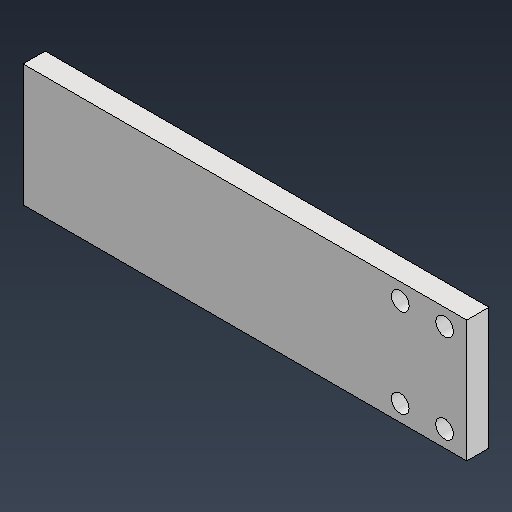
# Autodesk Inventor part: PLATE,HINGE,FRONT,INTAKE
Saved by Autodesk Inventor 2026 (Build 300175050, 175E)
## iProperties
Created: 2026-02-16
Part Number: PLATE,HINGE,FRONT,INTAKE
Material: Generic
Document SubType Name: Modeling
Designer: Jthib
Mass: 27.6453 g
Surface Area: 111.71 cm^2
Volume: 27.6453 cm^3
Density: 1 g/cm^3
Appearance: Default
Author: Jthib
Autodesk Inventor part; units mm, degrees
ref_plane "YZ Plane" through (0, 0, 0) normal (1, 0, 0) x (0, 1, 0)
ref_plane "XZ Plane" through (0, 0, 0) normal (0, 1, 0) x (-1, 0, 0)
ref_plane "XY Plane" through (0, 0, 0) normal (0, 0, 1) x (1, 0, 0)
sketch "Sketch1" plane through (0, 0, 0) normal (0, 0, 1) x (1, 0, 0)
  line L0 (63.5, -17.4625) -> (-63.5, -17.4625)
  line L1 (-63.5, -17.4625) -> (-63.5, 17.4625)
  line L2 (-63.5, 17.4625) -> (63.5, 17.4625)
  line L3 (63.5, 17.4625) -> (63.5, -17.4625)
  line L4 (63.5, -17.4625) -> (-63.5, 17.4625) construction
  line L5 (-63.5, -17.4625) -> (63.5, 17.4625) construction
  point P0 (0, 0)
  dimension "d0" = 34.925
  dimension "d1" = 127
  constraints: 12 end point, 2 midpoint, 2 parallel, 1 horizontal, 1 perpendicular
  measures "d0" distance of L2.end L0.start
  measures "d1" distance of L1.end L2.end
extrude "Extrusion1" add sketch "Sketch1" along normal mid plane 6.35
sketch "Sketch2" plane through (0, 0, 3.175) normal (0, 0, 1) x (1, 0, 0)
  line L0 (44.45, 12.7) -> (57.15, 12.7) construction
  line L1 (57.15, 12.7) -> (57.15, -12.7) construction
  line L2 (57.15, -12.7) -> (44.45, -12.7) construction
  line L3 (44.45, -12.7) -> (44.45, 12.7) construction
  line L4 (44.45, 12.7) -> (57.15, -12.7) construction
  line L5 (57.15, 12.7) -> (44.45, -12.7) construction
  line L6 (0, -24.4475) -> (0, 24.4475) construction
  line L7 (-88.9, 0) -> (88.9, 0) construction
  line L8 (63.5, -17.4625) -> (63.5, 17.4625) construction
  point P0 (0, 0)
  point P1 (50.8, 0)
  dimension "d4" = 25.4
  dimension "d5" = 12.7
  dimension "d14" = 12.7
  constraints: 12 end point, 2 midpoint, 2 parallel, 1 horizontal, 1 perpendicular, 1 point on line
  measures "d4" distance of L0.end L1.end
  measures "d5" distance of L1.end L2.end
  measures "d14" distance from line of L8 point (50.8, 0)
hole "Hole1" at (57.15, -12.7, 3.175) at (44.45, -12.7, 3.175) at (44.45, 12.7, 3.175) at (57.15, 12.7, 3.175) direction (0, 0, -1) diameter 5.1054 end through all clearance for "Flat Head Machine Screw (82)" size "#10" standard "Ansi Unified Screw Threads"
body "Solid1"
